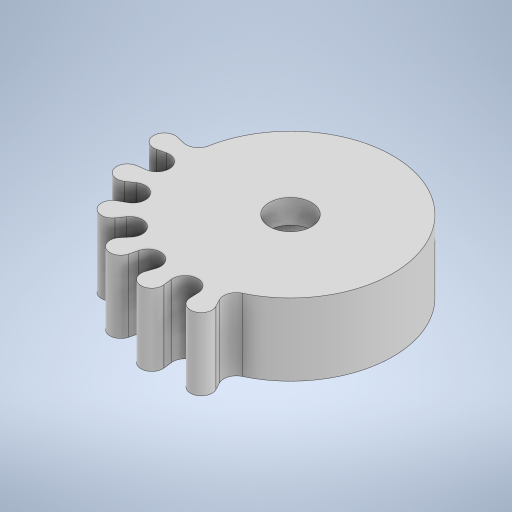
# Autodesk Inventor part: End_Effector_Claw_R_test
Saved by Autodesk Inventor 2023 (Build 270158000, 158)
## iProperties
Created: 2025-02-27
Part Number: End_Effector_Claw_R_test
Material: Generic
Document SubType Name: Modeling
Designer: Swoby
Density: 1 g/cm^3
Appearance: Default
Author: Swoby
Autodesk Inventor part; units mm, degrees
ref_plane "YZ Plane" through (0, 0, 0) normal (1, 0, 0) x (0, 1, 0)
ref_plane "XZ Plane" through (0, 0, 0) normal (0, 1, 0) x (-1, 0, 0)
ref_plane "XY Plane" through (0, 0, 0) normal (0, 0, 1) x (1, 0, 0)
sketch "Sketch1" plane through (0, 0, 0) normal (0, 1, 0) x (-1, 0, 0)
  line L0 (0, 0) -> (10, 0) construction
  circle A0 centre (10, 0) radius 8.5
  line L1 (0, 0) -> (-10, 0) construction
  circle A1 centre (-10, 0) radius 8.5 construction
  line L2 (10, 0) -> (21.547005, -20) construction
  line L3 (21.547005, -20) -> (21.547005, -40) construction
  line L4 (21.547005, -40) -> (0, -65.678721) construction
  line L5 (0, -69.606468) -> (0, -61.750975)
  arc A2 (0, -61.750975) -> (5.064556, -19.280066) centre (-15.413844, -38.375487) ccw
  line L6 (15.583183, -6.409217) -> (26.547005, -19.475392) construction
  line L7 (26.547005, -19.475392) -> (26.547005, -49.475392)
  line L8 (26.547005, -49.475392) -> (1.642788, -70.372512)
  arc A3 (4.416817, -6.409217) -> (5.064556, -19.280066) centre (12.37827, -12.460272) ccw
  arc A4 (5.064556, -19.280066) -> (0, -15) centre (-15.413844, -38.375487) ccw construction
  line L9 (15.583183, -6.409217) -> (4.416817, -6.409217) construction
  arc A5 (18.480915, 0.569287) -> (26.547005, -19.475392) centre (53.213867, 2.900761) ccw
  arc A6 (0, -69.606468) -> (1.642788, -70.372512) centre (1, -69.606468) ccw
  circle A7 centre (10, 0) radius 1.75
  circle A8 centre (10, 0) radius 3.4
  point P0 (0, -71.750975)
  dimension "d0" = 10
  dimension "d1" = 17
  dimension "d2" = 10
  dimension "d3" = 17
  dimension "d4" = 120
  dimension "d5" = 140
  dimension "d6" = 20
  dimension "d9" = 20
  dimension "d10" = 65.67872
  dimension "d11" = 10
  dimension "d12" = 15
  dimension "d14" = 50
  dimension "d15" = 5
  dimension "d16" = 30
  dimension "d18" = 10
  dimension "d19" = 28
  dimension "d20" = 1
  dimension "d52" = 3.5
  dimension "d53" = 6.8
  constraints: 20 end point, 13 point on circle, 9 centre point, 5 tangent, 4 coincident, 4 point on line, 3 horizontal, 3 vertical, 1 midpoint, 1 perpendicular
  measures "d0" distance of L0.start L0.end
  measures "d1" diameter of A0
  measures "d2" distance of L0.start L1.end
  measures "d3" diameter of A1
  measures "d4" angle of L0 L2
  measures "d5" angle of L3 L4
  measures "d6" distance of L2.end L3.end
  measures "d9" vertical distance of L2.start L2.end
  measures "d10" vertical distance of L4.end L0.end
  measures "d11" distance of point (0, -71.751) L5.end
  measures "d12" distance of L0.start A4.end
  measures "d14" angle of L6 L0
  measures "d15" distance between parallel lines of L3 L7
  measures "d16" distance of L6.end L7.end
  measures "d18" radius of A3
  measures "d19" radius of A2
  measures "d20" radius of A6
  measures "d52" diameter of A7
  measures "d53" diameter of A8
extrude "Extrusion1" add sketch "Sketch1" along normal blind 4 contours A0 | A0 A5 L7 L8 A6 L5 A2 A3 | A8
sketch "Sketch2" plane through (0, 4, 0) normal (0, 1, 0) x (1, 0, 0)
  circle A0 centre (10.329, 0) radius 8.5 construction
  arc A1 (0.297557, -0.876954) -> (1.399922, 0) centre (0.499922, 0) ccw
  arc A2 (-1.037626, -3.440333) -> (0.642818, -4.085395) centre (-0.197404, -3.762864) ccw construction
  circle A3 centre (-0.614315, -1.739534) radius 0.9 construction
  line L0 (-10, 0) -> (-18.428848, 0) construction
  line L1 (-10, 0) -> (0.499922, 0) construction
  line L2 (-10, 0) -> (-0.197404, -3.762864) construction
  arc A4 (-0.379229, -0.72078) -> (-1.642333, -1.549002) centre (-0.614315, -1.739534) ccw
  line L3 (-0.379229, -0.72078) -> (0.297557, -0.876954)
  line L4 (-0.759958, -2.774866) -> (-0.072032, -2.871639) construction
  arc A5 (-0.400078, 0) -> (0.297557, -0.876954) centre (0.499922, 0) ccw construction
  arc A6 (1.399922, 0) -> (0.37566, 0.89138) centre (0.499922, 0) ccw
  arc A7 (-0.072032, -2.871639) -> (-1.037626, -3.440333) centre (-0.197404, -3.762864) ccw construction
  arc A8 (0.642818, -4.085395) -> (-0.072032, -2.871639) centre (-0.197404, -3.762864) ccw construction
  arc A9 (0.37566, 0.89138) -> (-0.400078, 0) centre (0.499922, 0) ccw construction
  line L5 (-10, 0) -> (-0.614315, -1.739534) construction
  arc A10 (-18.480915, -0.569287) -> (-4.416817, 6.409217) centre (-10, 0) ccw
  arc A11 (-1.642333, -1.549002) -> (-0.759958, -2.774866) centre (-0.614315, -1.739534) ccw construction
  arc A12 (1.399922, 0) -> (0.297557, 0.876954) centre (0.499922, 0) ccw
  arc A13 (-1.642333, 1.549002) -> (-0.379229, 0.72078) centre (-0.614315, 1.739534) ccw
  line L6 (-0.379229, 0.72078) -> (0.297557, 0.876954)
  point P0 (0, 0)
  point P1 (0.37566, 0.89138)
  dimension "d47" = 84
  dimension "d23" = 10
  dimension "d24" = 10.329
  dimension "d26" = 17
  dimension "d36" = 1.8
  dimension "d37" = 1.8
  dimension "d38" = 1.8
  dimension "d39" = 10.49992
  dimension "d40" = 10.5
  dimension "d41" = 21
  dimension "d58" = 10.5
  dimension "d63" = 9.54553
  constraints: 23 point on circle, 14 end point, 13 centre point, 9 tangent, 7 point on line, 4 symmetric about line, 1 coincident, 1 collinear, 1 horizontal, 3 other
  measures "d23" distance of point (-10, 0) point (0, 0)
  measures "d24" distance of A0.centre point (0, 0)
  measures "d26" diameter of A0
  measures "d36" diameter of A1
  measures "d37" diameter of A2
  measures "d38" diameter of A3
  measures "d39" distance of point (-10, 0) L1.end
  measures "d40" distance of point (-10, 0) L2.end
  measures "d41" angle of L2 L1
  measures "d58" angle of L5 L1
  measures "d63" distance of L0.start L5.end
extrude "Extrusion2" add sketch "Sketch2" against normal up to surface (4 mm away)
pattern_circular "Circular Pattern1" count 6 over 105 about axis through (-10, 0, 0) along (0, -1, 0) of "Extrusion2"
mirror "Mirror1" about plane through (0, 0, 0) normal (1, 0, 0) remove original yes
sketch "Sketch3" plane through (26.547005, 0, -49.475392) normal (0, -1, 0) x (1, 0, 0)
  arc A0 (-22.130188, 43.066175) -> (-21.48245, 30.195327) centre (-14.168735, 37.01512) ccw
  arc A1 (-26.547005, -12.275582) -> (-21.48245, 30.195327) centre (-41.96085, 11.099905) ccw
  line L0 (-26.547005, -12.275582) -> (-26.547005, -20.131076)
  arc A2 (-26.547005, -20.131076) -> (-24.904218, -20.89712) centre (-25.547005, -20.131076) ccw
  line L1 (-24.904218, -20.89712) -> (0, 0)
  line L2 (0, 0) -> (0, 30)
  arc A3 (-8.066091, 50.044679) -> (0, 30) centre (26.666861, 52.376153) ccw
  arc A4 (-8.066091, 50.044679) -> (-12.887661, 57.147367) centre (-16.547005, 49.475392) ccw
  arc A5 (-13.360746, 58.581792) -> (-12.887661, 57.147367) centre (-12.43755, 58.091044) ccw
  line L3 (-13.034729, 59.195096) -> (-13.360746, 58.581792)
  arc A6 (-13.034729, 59.195096) -> (-14.728874, 59.649041) centre (-13.829426, 59.617538) ccw
  line L4 (-14.753187, 58.954895) -> (-14.728874, 59.649041)
  arc A7 (-16.835818, 59.118802) -> (-14.753187, 58.954895) centre (-15.798072, 58.991493) ccw
  line L5 (-16.751243, 59.808205) -> (-16.835818, 59.118802)
  arc A8 (-16.751243, 59.808205) -> (-18.495543, 59.624872) centre (-17.644546, 59.917794) ccw
  line L6 (-18.269481, 58.968118) -> (-18.495543, 59.624872)
  arc A9 (-20.272524, 58.37479) -> (-18.269481, 58.968118) centre (-19.258081, 58.627831) ccw
  line L7 (-20.440627, 59.048712) -> (-20.272524, 58.37479)
  arc A10 (-20.440627, 59.048712) -> (-22.00337, 58.252454) centre (-21.31387, 58.830891) ccw
  line L8 (-21.556964, 57.720335) -> (-22.00337, 58.252454)
  arc A11 (-23.214336, 56.448589) -> (-21.556964, 57.720335) centre (-22.357954, 57.048367) ccw
  line L9 (-23.612785, 57.017507) -> (-23.214336, 56.448589)
  arc A12 (-23.612785, 57.017507) -> (-24.786379, 55.714099) centre (-24.349968, 56.501211) ccw
  line L10 (-24.178928, 55.377301) -> (-24.786379, 55.714099)
  arc A13 (-25.270465, 53.596074) -> (-24.178928, 55.377301) centre (-24.685904, 54.462916) ccw
  line L11 (-25.846331, 53.984414) -> (-25.270465, 53.596074)
  arc A14 (-25.846331, 53.984414) -> (-26.474876, 52.346999) centre (-26.349527, 53.238228) ccw
  line L12 (-25.787074, 52.250262) -> (-26.474876, 52.346999)
  arc A15 (-26.167777, 50.196172) -> (-25.787074, 52.250262) centre (-25.932691, 51.214926) ccw
  line L13 (-26.844563, 50.352346) -> (-26.167777, 50.196172)
  arc A16 (-26.844563, 50.352346) -> (-26.844563, 48.598438) centre (-27.046927, 49.475392) ccw
  line L14 (-26.167777, 48.754612) -> (-26.844563, 48.598438)
  arc A17 (-24.904672, 47.92639) -> (-26.167777, 48.754612) centre (-25.932691, 47.735858) ccw
  arc A18 (-24.904672, 47.92639) -> (-22.130188, 43.066175) centre (-16.547005, 49.475392) ccw
  circle A19 centre (-16.547005, 49.475392) radius 1.75
  arc A20 (-13.033293, 50.785477) -> (-19.80916, 47.625838) centre (-16.547005, 49.475392) ccw
  line L15 (-16.547005, 49.475392) -> (-9.890768, 35.201044) construction
  arc A21 (-12.065537, 33.968009) -> (-7.548293, 36.074434) centre (-9.890768, 35.201044) ccw
  line L16 (-13.033293, 50.785477) -> (-7.548293, 36.074434)
  line L17 (-19.80916, 47.625838) -> (-12.065537, 33.968009)
  line L18 (-16.526291, 49.430971) -> (-18.131824, 52.874046) construction
  line L19 (-9.890768, 35.201044) -> (-8.834222, 32.935275) construction
  arc A22 (-14.962187, 46.076738) -> (-13.033293, 50.785477) centre (-16.547005, 49.475392) ccw construction
  arc A23 (-19.80916, 47.625838) -> (-14.962187, 46.076738) centre (-16.547005, 49.475392) ccw construction
  arc A24 (-10.947313, 37.466814) -> (-12.065537, 33.968009) centre (-9.890768, 35.201044) ccw construction
  arc A25 (-7.548293, 36.074434) -> (-10.947313, 37.466814) centre (-9.890768, 35.201044) ccw construction
  point P0 (-26.547005, 49.475392)
  dimension "d67" = 7.5
  dimension "d68" = 25
  dimension "d69" = 22
  dimension "d70" = 5
  constraints: 16 point on circle, 10 end point, 8 tangent, 6 centre point, 3 point on line, 2 coincident, 2 collinear
  measures "d67" diameter of A20
  measures "d68" angle of L2 L15
  measures "d69" distance of L19.end L18.end
  measures "d70" diameter of A21
sketch "Sketch4" plane through (-0.499922, 4, 0) normal (0, 1, 0) x (1, 0, 0)
  arc A0 (5.564478, 19.280066) -> (4.916739, 6.409217) centre (12.878192, 12.460272) ccw
  arc A1 (4.916739, 6.409217) -> (2.142255, 1.549002) centre (10.499922, 0) ccw
  arc A2 (0.87915, 0.72078) -> (2.142255, 1.549002) centre (1.114237, 1.739534) ccw
  line L0 (0.202365, 0.876954) -> (0.87915, 0.72078)
  arc A3 (0.202365, 0.876954) -> (0.202365, -0.876954) centre (0, 0) ccw
  line L1 (0.87915, -0.72078) -> (0.202365, -0.876954)
  arc A4 (1.259854, -2.77487) -> (0.87915, -0.72078) centre (1.114237, -1.739534) ccw
  line L2 (0.572052, -2.871607) -> (1.259854, -2.77487)
  arc A5 (0.572052, -2.871607) -> (1.200596, -4.509022) centre (0.6974, -3.762836) ccw
  line L3 (1.776463, -4.120682) -> (1.200596, -4.509022)
  arc A6 (2.867999, -5.901909) -> (1.776463, -4.120682) centre (2.361023, -4.987524) ccw
  line L4 (2.260549, -6.238707) -> (2.867999, -5.901909)
  arc A7 (2.260549, -6.238707) -> (3.434142, -7.542115) centre (2.696959, -7.025819) ccw
  line L5 (3.832591, -6.973197) -> (3.434142, -7.542115)
  arc A8 (5.489963, -8.244943) -> (3.832591, -6.973197) centre (4.688974, -7.572975) ccw
  line L6 (5.043557, -8.777062) -> (5.489963, -8.244943)
  arc A9 (5.043557, -8.777062) -> (6.606301, -9.57332) centre (5.733057, -9.355499) ccw
  line L7 (6.774403, -8.899397) -> (6.606301, -9.57332)
  arc A10 (8.777446, -9.492726) -> (6.774403, -8.899397) centre (7.788846, -9.152439) ccw
  line L8 (8.551384, -10.14948) -> (8.777446, -9.492726)
  arc A11 (8.551384, -10.14948) -> (10.295684, -10.332813) centre (9.402381, -10.442402) ccw
  line L9 (10.211109, -9.64341) -> (10.295684, -10.332813)
  arc A12 (12.293741, -9.479503) -> (10.211109, -9.64341) centre (11.248855, -9.5161) ccw
  line L10 (12.318053, -10.173649) -> (12.293741, -9.479503)
  arc A13 (12.318053, -10.173649) -> (14.012199, -9.719704) centre (13.217502, -10.142146) ccw
  line L11 (13.686181, -9.1064) -> (14.012199, -9.719704)
  arc A14 (14.159266, -7.671975) -> (13.686181, -9.1064) centre (14.609377, -8.615651) ccw
  arc A15 (14.159266, -7.671975) -> (18.980837, -0.569287) centre (10.499922, 0) ccw
  arc A16 (27.046927, 19.475392) -> (18.980837, -0.569287) centre (53.713789, -2.900761) ccw
  line L12 (27.046927, 49.475392) -> (27.046927, 19.475392)
  line L13 (2.14271, 70.372512) -> (27.046927, 49.475392)
  arc A17 (2.14271, 70.372512) -> (0.499922, 69.606468) centre (1.499922, 69.606468) ccw
  line L14 (0.499922, 61.750975) -> (0.499922, 69.606468)
  arc A18 (5.564478, 19.280066) -> (0.499922, 61.750975) centre (-14.913922, 38.375487) ccw
  circle A19 centre (10.499922, 0) radius 1.75
  line L15 (4.916739, 6.409217) -> (16.659694, 26.748611)
  arc A20 (27.046927, 19.475392) -> (27.046927, 27.657377) centre (22.171473, 23.566384) ccw construction
  arc A21 (27.046927, 27.657377) -> (16.659694, 26.748611) centre (22.171473, 23.566384) ccw
  point P0 (0.499922, 0)
  dimension "d72" = 150
  constraints: 4 point on circle, 3 tangent, 2 centre point, 2 end point, 1 point on line
  measures "d72" angle of L15 L12
extrude "Extrusion5" add sketch "Sketch4" along normal blind 2 contours L15 A21 L12 A16 A15 A14 L11 A13 L10 A12 L9 A11 L8 A10 L7 A9 L6 A8 L5 A7 L4 A6 L3 A5 L2 A4 L1 A3 L0 A2 A1
extrude "Extrusion6" cut sketch "Sketch3" against normal blind 4 contours L16 A21 L17 A20
chamfer "Chamfer1" distance 1 angle 45 12 edges at (12.3892, 0, -41.6909) (2.3909, 0, -12.9629) (14.0949, 0, -59.924) (0.5774, 0, -70.5128) (0, 0, -65.6787) (26.547, 0, -34.4754) (26.547, 4, -38.5664) (14.0949, 4, -59.924) (0.5774, 4, -70.5128) (0, 4, -65.6787) (12.3892, 4, -41.6909) (2.3909, 4, -12.9629)
sketch "Sketch5" plane through (-0.499922, 6, 0) normal (0, 1, 0) x (1, 0, 0)
  arc A0 (4.916739, 6.409217) -> (2.142255, 1.549002) centre (10.499922, 0) ccw
  arc A1 (0.87915, 0.72078) -> (2.142255, 1.549002) centre (1.114237, 1.739534) ccw
  line L0 (0.87915, 0.72078) -> (0.202365, 0.876954)
  arc A2 (0.202365, 0.876954) -> (0.202365, -0.876954) centre (0, 0) ccw
  line L1 (0.202365, -0.876954) -> (0.87915, -0.72078)
  arc A3 (1.259854, -2.77487) -> (0.87915, -0.72078) centre (1.114237, -1.739534) ccw
  line L2 (1.259854, -2.77487) -> (0.572052, -2.871607)
  arc A4 (0.572052, -2.871607) -> (1.200596, -4.509022) centre (0.6974, -3.762836) ccw
  line L3 (1.200596, -4.509022) -> (1.776463, -4.120682)
  arc A5 (2.867999, -5.901909) -> (1.776463, -4.120682) centre (2.361023, -4.987524) ccw
  line L4 (2.867999, -5.901909) -> (2.260549, -6.238707)
  arc A6 (2.260549, -6.238707) -> (3.434142, -7.542115) centre (2.696959, -7.025819) ccw
  line L5 (3.434142, -7.542115) -> (3.832591, -6.973197)
  arc A7 (5.489963, -8.244943) -> (3.832591, -6.973197) centre (4.688974, -7.572975) ccw
  line L6 (5.489963, -8.244943) -> (5.043557, -8.777062)
  arc A8 (5.043557, -8.777062) -> (6.606301, -9.57332) centre (5.733057, -9.355499) ccw
  line L7 (6.606301, -9.57332) -> (6.774403, -8.899397)
  arc A9 (8.777446, -9.492726) -> (6.774403, -8.899397) centre (7.788846, -9.152439) ccw
  line L8 (8.777446, -9.492726) -> (8.551384, -10.14948)
  arc A10 (8.551384, -10.14948) -> (10.295684, -10.332813) centre (9.402381, -10.442402) ccw
  line L9 (10.295684, -10.332813) -> (10.211109, -9.64341)
  arc A11 (12.293741, -9.479503) -> (10.211109, -9.64341) centre (11.248855, -9.5161) ccw
  line L10 (12.293741, -9.479503) -> (12.318053, -10.173649)
  arc A12 (12.318053, -10.173649) -> (14.012199, -9.719704) centre (13.217502, -10.142146) ccw
  line L11 (14.012199, -9.719704) -> (13.686181, -9.1064)
  arc A13 (14.159266, -7.671975) -> (13.686181, -9.1064) centre (14.609377, -8.615651) ccw
  arc A14 (14.159266, -7.671975) -> (18.980837, -0.569287) centre (10.499922, 0) ccw
  arc A15 (27.046927, 19.475392) -> (18.980837, -0.569287) centre (53.713789, -2.900761) ccw
  line L12 (27.046927, 19.475392) -> (27.046927, 27.657377)
  arc A16 (27.046927, 27.657377) -> (16.659694, 26.748611) centre (22.171473, 23.566384) ccw
  line L13 (16.659694, 26.748611) -> (4.916739, 6.409217)
  circle A17 centre (10.499922, 0) radius 1.75
  arc A18 (2.142255, -1.549002) -> (14.159266, -7.671975) centre (10.499922, 0) ccw construction
  arc A19 (2.142255, 1.549002) -> (2.142255, -1.549002) centre (10.499922, 0) ccw construction
  arc A20 (14.159266, -7.671975) -> (2.142255, 1.549002) centre (10.499922, 0) ccw
  point P0 (0.499922, 0)
  point P1 (18.980837, -0.569287)
  point P2 (4.916739, 6.409217)
  constraints: 9 point on circle, 3 centre point, 1 coincident, 1 concentric
extrude "Extrusion7" cut sketch "Sketch5" against normal through all contours A20 A14 A13 L11 A12 L10 A11 L9 A10 L8 A9 L7 A8 L6 A7 L5 A6 L4 A5 L3 A4 L2 A3 L1 A2 L0 A1 A0 keep common part
equation "\"d3\" = d1"
equation "\"d26\" = 2 * d25"
equation "\"d58\" = 0.5 * d41"
equation "\"d25\" = 8.5"
body "Solid1"
